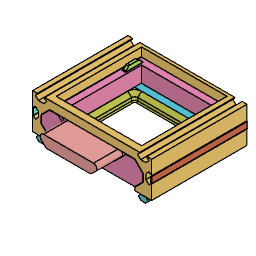
gridfinity_drawer (Autodesk Fusion 360 design; units mm, degrees)
part number: 2026-01-11-15-52-53-317
part number: 2026-01-11-15-53-28-948
part number: 2026-01-11-15-53-37-939
part number: 2026-01-11-16-03-17-954
part number: 2026-01-11-18-22-58-266
part number: 2026-01-11-18-42-20-558
part number: 2026-01-11-19-37-17-001
part number: 2026-01-13-18-50-05-171
part number: 2026-01-13-18-58-14-799
part number: 2026-01-13-19-49-23-785
part number: 2026-01-14-18-30-10-930
part number: 2026-01-14-18-30-21-173
part number: 2026-01-14-18-30-45-681
part number: 2026-01-17-12-17-04-401
part number: 2026-01-17-12-24-58-643
part number: 2026-01-17-12-34-27-194
part number: 2026-01-17-12-59-30-630
Autodesk Fusion 360 part; units mm, degrees
note: some values were not read from the file. Chosen so that the rebuilt part matches the saved one: which bodies a step acts on; that a step has no effect; a side. Set by a fixed rule: which sketch regions a step uses.
(part 1 of 2)
sketch "Schizzo1" plane through (0, 0, 0) normal (0, 0, 1) x (1, 0, 0) in component "baseplate"
  line L0 (4, 0) -> (38, 0)
  line L1 (42, 4) -> (42, 38)
  line L2 (38, 42) -> (4, 42)
  line L3 (0, 38) -> (0, 4)
  arc A0 (4, 42) -> (0, 38) centre (4, 38) ccw
  arc A1 (42, 38) -> (38, 42) centre (38, 38) ccw
  arc A2 (0, 4) -> (4, 0) centre (4, 4) ccw
  arc A3 (38, 0) -> (42, 4) centre (38, 4) ccw
  line L4 (0, 0) -> (42, 0)
  line L5 (42, 0) -> (42, 42)
  line L6 (42, 42) -> (0, 42)
  line L7 (0, 42) -> (0, 0)
  point P0 (42, 0)
  point P1 (0, 42)
  dimension "d3" = 42
  dimension "d4" = 42
  dimension "d5" = 4
  dimension "d6" = 4
  dimension "d7" = 4
  dimension "d8" = 4
  dimension "d9" = 42
  dimension "d10" = 42
  constraint horizontal L0
  constraint vertical L1
  constraint horizontal L2
  constraint vertical L3
  constraint coincident L4.start L7.end
  constraint coincident P1 L2
  constraint coincident P1 L3
  constraint tangent L2 A0
  constraint tangent L3 A0
  constraint tangent L2 A1
  constraint tangent L1 A1
  constraint coincident L4.start L3
  constraint coincident L4.start L0
  constraint tangent L3 A2
  constraint tangent L0 A2
  constraint coincident P0 L1
  constraint coincident P0 L0
  constraint tangent L1 A3
  constraint tangent L0 A3
  constraint horizontal L4
  constraint vertical L5
  constraint horizontal L6
  constraint vertical L7
  measures "d3" distance of L4.start P0
  measures "d4" distance of L4.start L6.end
  measures "d5" radius of A0
  measures "d6" radius of A1
  measures "d7" radius of A2
  measures "d8" radius of A3
  measures "d9" distance of L4.start P0
  measures "d10" distance of L4.start P1
ref_plane "Piano di lavoro1" through (21, 0, 0) normal (0, -1, 0) x (1, 0, 0) in component "baseplate"
ref_plane "Piano di lavoro2" through (21, 42, 0) normal (0, 1, 0) x (-1, 0, 0) in component "baseplate"
ref_plane "Piano di lavoro3" through (21, 21, 0) normal (0, 1, 0) x (-1, 0, 0) in component "baseplate"
sketch "Schizzo2" plane through (0, 21, 0) normal (0, 1, 0) x (1, 0, 0) in component "baseplate"
  line L0 (0, 0) -> (2.85, 0)
  line L1 (2.85, 0) -> (2.15, -0.7)
  line L2 (2.85, 0) -> (0, 0) construction
  line L3 (2.15, -0.7) -> (2.15, -2.5)
  line L4 (2.15, -2.5) -> (0, -4.65)
  line L5 (2.15, -2.5) -> (0, -2.5) construction
  line L6 (0, 0) -> (0, -4.65)
  dimension "d13" = 2.85
  dimension "d14" = 45
  dimension "d15" = 1.8
  dimension "d16" = 45
  dimension "d17" = 0.7
  dimension "d18" = 2.15
  dimension "d19" = 4.65
  constraint coincident L0.start L2.end
  constraint horizontal L0
  constraint horizontal L2
  constraint vertical L3
  constraint horizontal L5
  constraint coincident L5.end L6
  measures "d13" distance of L0.start L0.end
  measures "d14" angle of L1 L2
  measures "d15" distance of L1.end L3.end
  measures "d16" angle of L4 L5
  measures "d17" distance of L1.end L2
  measures "d18" distance of L4.end L5
  measures "d19" distance of L4.end L0.start
sweep "Sweep1" add profiles "Schizzo2" path "Schizzo1" along A2 L0 A3 L1 A1 L2 A0 L3 section 1 makes body 1 in component "baseplate"
extrude "Estrusione1" add sketch "Schizzo1" along normal blind 4.65 contours A2 L4 L7 | A3 L4 L5 | A0 L6 L7 | A1 L5 L6 bodies 1 in component "baseplate"
pattern_linear "Serie R1" [no effect] in component "baseplate"
sketch "Schizzo1 (2)" plane through (0, 0, 0) normal (0, 0, 1) x (1, 0, 0) in component "offset"
  line L0 (0, 0) -> (42, 0)
  line L1 (42, 0) -> (42, 42)
  line L2 (42, 42) -> (0, 42)
  line L3 (0, 42) -> (0, 0)
  line L4 (42.2, 46) -> (-0.2, 46)
  line L5 (42.2, 0) -> (42.2, 46)
  line L6 (-0.2, 46) -> (-0.2, 0)
  line L7 (0, 0) -> (-0.2, 0)
  line L8 (42, 0) -> (42.2, 0)
  dimension "d87" = 42
  dimension "d88" = 42
  dimension "d89" = 4
  dimension "d90" = 0.2
  dimension "d91" = 0.2
  constraint horizontal L0
  constraint vertical L1
  constraint horizontal L2
  constraint vertical L3
  constraint coincident L0.start L3.end
  constraint perpendicular L6 L7
  constraint perpendicular L5 L8
  constraint coincident L4 L6.start
  constraint coincident L4 L5.end
  constraint coincident L4.start L5
  constraint coincident L4.end L6
  measures "d87" distance of L0.start L0.end
  measures "d88" distance of L0.start L2.end
extrude "Estrusione3" add sketch "Schizzo1 (2)" along normal blind 4.65 separate body contours L1 L2 L3 L4 L5 L6 L7 L8 makes body 2 in component "offset"
sketch "Schizzo1 (3)" plane through (0, 0, 0) normal (0, 0, 1) x (1, 0, 0) in component "walls"
  line L0 (-0.2, 46) -> (42.2, 46) construction
  line L1 (42.2, 46) -> (42.2, 0) construction
  line L2 (42.2, 0) -> (-0.2, 0) construction
  line L3 (-0.2, 0) -> (-0.2, 46) construction
  line L4 (0, 46) -> (0, 0)
  line L5 (0, 46) -> (-8.8, 46)
  line L6 (-8.8, 46) -> (-8.8, 0)
  line L7 (-8.8, 0) -> (0, 0)
  line L8 (0, 0) -> (0, 46)
  line L9 (21, 46) -> (21, 0) construction
  line L10 (42, 46) -> (50.8, 46)
  line L11 (42, 0) -> (42, 46)
  line L12 (50.8, 46) -> (50.8, 0)
  line L13 (50.8, 0) -> (42, 0)
  line L14 (-8.8, 46) -> (50.8, 46)
  line L15 (50.8, 46) -> (50.8, 50)
  line L16 (50.8, 50) -> (-8.8, 50)
  line L17 (-8.8, 50) -> (-8.8, 46)
  line L18 (-0.2, 23) -> (42.2, 23) construction
  line L19 (50.8, -4) -> (-8.8, -4)
  line L20 (-8.8, -4) -> (-8.8, 0)
  line L21 (-8.8, 0) -> (50.8, 0)
  line L22 (50.8, 0) -> (50.8, -4)
  point P0 (-0.2, 46)
  point P1 (42.2, 0)
  dimension "d107" = 0.2
  dimension "d108" = 8.8
  dimension "d109" = 4
  constraint horizontal L0
  constraint vertical L1
  constraint horizontal L2
  constraint vertical L3
  constraint coincident P1 L1.end
  constraint coincident P0 L0.start
  constraint coincident L0 L4.start
  constraint perpendicular L2 L4
  constraint coincident L2 L4.end
  constraint horizontal L5
  constraint vertical L6
  constraint horizontal L7
  constraint vertical L8
  constraint midpoint L0 L9.start
  constraint midpoint L2 L9.end
  constraint symmetric L4.start L9 L10.start
  constraint symmetric L5.end L9 L10.end
  constraint symmetric L6.end L9 L12.end
  constraint symmetric L4.end L9 L11.start
  constraint horizontal L14
  constraint vertical L15
  constraint horizontal L16
  constraint vertical L17
  constraint coincident L12 L10.end
  constraint midpoint L3 L18.start
  constraint midpoint L1 L18.end
  constraint symmetric L5.end L18 L6.end
  constraint symmetric L10.end L18 L12.end
  constraint symmetric L15.end L18 L19.start
  constraint symmetric L16.end L18 L19.end
  measures "d107" distance of L3 L4
  measures "d108" distance of L4.start L5.end
  measures "d109" distance of L5.end L16.end
extrude "Estrusione1'" add sketch "Schizzo1 (3)" along normal blind 14 separate body contours L4 L5 L6 L7 L8 L14 L21 | L5 L10 L14 L15 L16 L17 | L7 L13 L19 L20 L21 L22 | L10 L11 L12 L13 L14 L21 makes body 3 in component "walls"
sketch "Schizzo2 (2)" plane through (0, -4, 0) normal (0, -1, 0) x (1, 0, 0) in component "walls"
  line L0 (-8.8, 0) -> (50.8, 0)
  line L1 (50.8, 0) -> (50.8, 14)
  line L2 (50.8, 14) -> (-8.8, 14)
  line L3 (-8.8, 14) -> (-8.8, 0)
  line L4 (21, 14) -> (21, 0) construction
  line L5 (-8.8, 7) -> (50.8, 7) construction
  line L6 (-4, 14) -> (-8.8, 9.2)
  line L7 (-4, 14) -> (-8.8, 14) construction
  line L8 (-4, 0) -> (-8.8, 4.8)
  line L9 (46, 14) -> (50.8, 9.2)
  line L10 (46, 0) -> (50.8, 4.8)
  dimension "d112" = 45
  dimension "d113" = 4.8
  constraint midpoint L2 L4.start
  constraint midpoint L0 L4.end
  constraint midpoint L3 L5.start
  constraint midpoint L1 L5.end
  constraint horizontal L7
  constraint coincident L2 L6.start
  constraint coincident L3 L6.end
  constraint coincident L3 L2.end
  constraint symmetric L5 L6.start L8.start
  constraint symmetric L5 L6.end L8.end
  constraint symmetric L4 L6.start L9.start
  constraint symmetric L4 L6.end L9.end
  constraint symmetric L4 L8.start L10.start
  constraint symmetric L4 L8.end L10.end
  measures "d112" angle of L6 L7
  measures "d113" distance of L3 L6.start
extrude "Estrusione2" cut sketch "Schizzo2 (2)" against normal up to surface (54 mm away) contours L0 L3 L8 | L0 L1 L10 | L2 L3 L6 | L1 L2 L9 bodies 3 in component "walls"
ref_plane "Piano di lavoro1" through (21, 23, 4.65) normal (0, 0, 1) x (1, 0, 0) in component "dividers"
sketch "Schizzo1 (4)" plane through (0, 0, 4.65) normal (0, 0, 1) x (1, 0, 0) in component "dividers"
  line L0 (42.2, 46) -> (-0.2, 46) construction
  line L1 (-1.8, 46) -> (0, 46)
  line L2 (0, 46) -> (0, 0)
  line L3 (0, 0) -> (-1.8, 0)
  line L4 (-1.8, 0) -> (-1.8, 46)
  line L5 (21, 46) -> (21, 34) construction
  line L6 (42, 46) -> (42, 0)
  line L7 (43.8, 46) -> (42, 46)
  line L8 (43.8, 0) -> (43.8, 46)
  line L9 (42, 0) -> (43.8, 0)
  line L10 (-1.8, 43.8) -> (43.8, 43.8)
  line L11 (43.8, 43.8) -> (43.8, 42)
  line L12 (43.8, 42) -> (-1.8, 42)
  line L13 (-1.8, 42) -> (-1.8, 43.8)
  point P0 (0, 42)
  dimension "d126" = 1.8
  dimension "d127" = 1.8
  constraint horizontal L1
  constraint vertical L2
  constraint horizontal L3
  constraint vertical L4
  constraint coincident L0 L1.end
  constraint coincident P0 L2
  constraint coincident L2.end L3.start
  constraint midpoint L0 L5.start
  constraint perpendicular L0 L5
  constraint symmetric L1.start L5 L7.start
  constraint symmetric L1.end L5 L6.start
  constraint symmetric L2.end L5 L6.end
  constraint symmetric L3.end L5 L8.start
  constraint horizontal L10
  constraint vertical L11
  constraint horizontal L12
  constraint vertical L13
  constraint coincident L4 L12.end
  constraint coincident P0 L12
  constraint coincident L8 L11.end
  measures "d126" distance of L1.start L1.end
  measures "d127" distance of L10.end L11.end
extrude "Estrusione2'" add sketch "Schizzo1 (4)" along normal blind 9.35 separate body contours L1 L2 L4 L10 | L2 L4 L10 L12 L13 | L2 L3 L4 L12 | L6 L8 L10 L11 L12 | L6 L7 L8 L10 | L6 L8 L9 L12 makes body 4 at (0, 30.6667, 7.7667) makes body 5 at (43.8, 30.6667, 10.8833) in component "dividers"
extrude "Estrusione3'" add sketch "Schizzo1 (4)" along normal blind 9.35 separate body contours L2 L6 L10 L12 makes body 6 in component "dividers"
extrude "Estrusione4" cut 1 faces at (0, 43.2, 7.7667) along direction (1, 0, 0) blind 1 on bodies 6 bodies 6 in component "dividers"
extrude "Estrusione5" cut 1 faces at (42, 43.2, 10.8833) along direction (-1, 0, 0) blind 1 on bodies 6 bodies 6 in component "dividers"
extrude "Estrusione6" add 1 faces at (1, 43.2, 7.7667) along direction (-1, 0, 0) up to surface (1 mm away) on bodies 6 bodies 6 in component "dividers"
extrude "Estrusione7" add 1 faces at (41, 43.2, 10.8833) along direction (1, 0, 0) up to surface (1 mm away) on bodies 6 bodies 6 in component "dividers"
ref_plane "Piano di lavoro1" through (21, -2, 7) normal (0, -1, 0) x (1, 0, 0) in component " handle recess"
sketch "Schizzo1 (5)" plane through (0, -2, 0) normal (0, -1, 0) x (-1, 0, 0) in component " handle recess"
  line L0 (4, -14) -> (-46, -14) construction
  line L1 (-46, -14) -> (-46, 0) construction
  line L2 (-46, 0) -> (4, 0) construction
  line L3 (4, 0) -> (4, -14) construction
  line L4 (-21, -14) -> (-21, 0) construction
  line L5 (-1, -14) -> (-7.75, -7.25)
  line L6 (-1, -14) -> (-9.2299, -14) construction
  line L7 (-41, -14) -> (-34.25, -7.25)
  line L8 (-7.75, -7.25) -> (-34.25, -7.25)
  line L9 (-41, -14) -> (-1, -14)
  line L10 (-21, -14) -> (-21, -24) construction
  line L11 (-21, -24) -> (-16, -24) construction
  line L12 (-1, -14) -> (9, -24)
  line L13 (-1, -14) -> (5.2856, -14) construction
  line L14 (-41, -14) -> (-51, -24)
  line L15 (-41, -14) -> (-49.4329, -14) construction
  point P0 (4, -14)
  point P1 (-46, 0)
  dimension "d142" = 45
  dimension "d143" = 20
  dimension "d144" = 6.75
  dimension "d145" = 10
  dimension "d146" = 5
  dimension "d147" = 45
  dimension "d148" = 45
  constraint horizontal L0
  constraint vertical L1
  constraint horizontal L2
  constraint vertical L3
  constraint coincident P1 L1.end
  constraint coincident P0 L0.start
  constraint midpoint L0 L4.start
  constraint midpoint L2 L4.end
  constraint horizontal L6
  constraint coincident L0 L5.start
  constraint symmetric L4 L5.start L7.start
  constraint symmetric L4 L5.end L7.end
  constraint perpendicular L0 L10
  constraint perpendicular L10 L11
  constraint horizontal L13
  constraint coincident L11 L12.end
  constraint horizontal L15
  constraint coincident L11 L14.end
  measures "d142" angle of L5 L6
  measures "d143" distance of L4.start L5.start
  measures "d144" distance of L5.end L6
  measures "d145" distance of L4.start L10.end
  measures "d146" distance of L10.end L11.end
  measures "d147" angle of L12 L13
  measures "d148" angle of L14 L15
ref_plane "Piano di lavoro2" through (-9, -2, 24) normal (-0.707107, 0, 0.707107) x (0, -1, 0) in component " handle recess"
sketch "Schizzo2 (3)" plane through (-9, -2, 24) normal (-0.707107, 0, 0.707107) x (0, -1, 0) in component " handle recess"
  line L0 (0.9, -2.4) -> (-0.9, -2.4)
  line L1 (-0.9, -2.4) -> (-0.9, 2.4)
  line L2 (-0.9, 2.4) -> (0.9, 2.4)
  line L3 (0.9, 2.4) -> (0.9, -2.4)
  line L4 (0.9, -2.4) -> (-0.9, 2.4) construction
  line L5 (-0.9, -2.4) -> (0.9, 2.4) construction
  dimension "d150" = 1.8
  dimension "d151" = 4.8
  constraint horizontal L0
  constraint perpendicular L0 L1
  constraint parallel L0 L2
  constraint parallel L1 L3
  constraint coincident L4 origin
  constraint coincident L5 origin
  measures "d150" distance of L1.end L2.end
  measures "d151" distance of L0.start L2.end
extrude "Estrusione3''" cut sketch "Schizzo1 (5)" along normal mid plane 4 bodies 3 in component "walls"
sweep "Sweep1'" cut profiles "Schizzo2 (3)" path "Schizzo1 (5)" along L14 L7 L8 L5 L12 section 1 bodies 3 in component "walls"
ref_plane "Piano di lavoro1" through (21, 23, 14) normal (0, 0, 1) x (1, 0, 0) in component "walls"
sketch "Schizzo3" plane through (0, 0, 14) normal (0, 0, 1) x (1, 0, 0) in component "walls"
  line L0 (-4, 50) -> (46, 50) construction
  line L1 (46, 50) -> (46, -4) construction
  line L2 (46, -4) -> (-4, -4) construction
  line L3 (-4, -4) -> (-4, 50) construction
  line L4 (21, 50) -> (21, -4) construction
  line L5 (-3, 48) -> (-1, 48)
  line L6 (-1, 48) -> (-1, 37.6)
  line L7 (-1, 37.6) -> (-3, 37.6)
  line L8 (-3, 37.6) -> (-3, 48)
  line L9 (43, 48) -> (43, 37.6)
  line L10 (45, 48) -> (43, 48)
  line L11 (45, 37.6) -> (45, 48)
  line L12 (43, 37.6) -> (45, 37.6)
  point P0 (-4, 50)
  point P1 (46, -4)
  dimension "d161" = 2
  dimension "d162" = 2
  dimension "d163" = 1
  dimension "d164" = 10.4
  constraint horizontal L0
  constraint vertical L1
  constraint horizontal L2
  constraint vertical L3
  constraint coincident P1 L1.end
  constraint coincident P0 L0.start
  constraint midpoint L0 L4.start
  constraint midpoint L2 L4.end
  constraint horizontal L5
  constraint vertical L6
  constraint horizontal L7
  constraint vertical L8
  constraint symmetric L4 L5.start L10.start
  constraint symmetric L4 L5.end L9.start
  constraint symmetric L4 L6.end L9.end
  constraint symmetric L4 L7.end L11.start
  measures "d161" distance of L0 L5
  measures "d162" distance of L5.start L5.end
  measures "d163" distance of L3 L8
  measures "d164" distance of L5.start L7.end
extrude "Estrusione4'" cut sketch "Schizzo3" against normal blind 10.4 bodies 3 in component "walls"
ref_plane "Piano di lavoro1" through (21, -1.1, 14) normal (0, -1, 0) x (-0.707107, 0, -0.707107) in component "handle"
sketch "Schizzo1 (6)" plane through (0, -1.1, 0) normal (0, -1, 0) x (-1, 0, 0) in component "handle"
  line L0 (2.3941, -14) -> (-6.7559, -4.85)
  line L1 (-6.7559, -4.85) -> (-35.2441, -4.85)
  line L2 (-35.2441, -4.85) -> (-44.3941, -14)
  line L3 (-44.3941, -14) -> (2.3941, -14)
  point P0 (2.3941, -14)
  point P1 (-6.7559, -4.85)
  point P2 (-35.2441, -4.85)
  point P3 (-44.3941, -14)
  constraint coincident P0 L0.start
  constraint coincident P1 L0.end
  constraint coincident P2 L1.end
  constraint coincident P3 L2.end
extrude "Estrusione1''" add sketch "Schizzo1 (6)" along normal blind 1.8 separate body makes body 7 in component "handle"
extrude "Estrusione6'" cut 1 faces at (13.202, -2.3, 14) along direction (0, 0, -1) blind 0.2 on bodies 7 bodies 7 in component "handle"
fillet "Raccordo2" radius 0.8 4 edges at (-2.1941, -2, 13.8) (6.7559, -2, 4.85) (35.2441, -2, 4.85) (44.1941, -2, 13.8) on bodies 7 in component "handle"
sketch "Schizzo3 (2)" plane through (0, -2.9, 0) normal (0, -1, 0) x (1, 0, 0) in component "handle"
  line L0 (-0.8284, 12.4343) -> (6.5216, 5.0843)
  line L1 (7.0873, 4.85) -> (34.9127, 4.85)
  line L2 (35.4784, 5.0843) -> (42.8284, 12.4343)
  line L3 (1, 14) -> (7.75, 7.25)
  line L4 (7.75, 7.25) -> (34.25, 7.25)
  line L5 (34.25, 7.25) -> (41, 14)
  line L6 (41, 14) -> (1, 14)
  line L7 (1.4828, 13.8) -> (7.8328, 7.45)
  line L8 (7.8328, 7.45) -> (34.1672, 7.45)
  line L9 (34.1672, 7.45) -> (40.5172, 13.8)
  line L10 (40.5172, 13.8) -> (1.4828, 13.8)
  arc A0 (42.8284, 12.4343) -> (42.2627, 13.8) centre (42.2627, 13) ccw
  line L11 (42.2627, 13.8) -> (-0.2627, 13.8)
  arc A1 (-0.2627, 13.8) -> (-0.8284, 12.4343) centre (-0.2627, 13) ccw
  arc A2 (6.5216, 5.0843) -> (7.0873, 4.85) centre (7.0873, 5.65) ccw
  arc A3 (34.9127, 4.85) -> (35.4784, 5.0843) centre (34.9127, 5.65) ccw
  point P0 (1, 14)
  point P1 (7.75, 7.25)
  point P2 (34.25, 7.25)
  point P3 (41, 14)
  dimension "d173" = -0.2
  constraint coincident P0 L3.start
  constraint coincident P1 L3.end
  constraint coincident P2 L4.end
  constraint coincident P3 L5.end
extrude "Estrusione4''" add sketch "Schizzo3 (2)" along normal blind 15 separate body contours L7 L8 L9 L10 L11 makes body 8 in component "handle"
fillet "Raccordo1" radius 2 4 edges at (1.4828, -10.4, 13.8) (7.8328, -10.4, 7.45) (34.1672, -10.4, 7.45) (40.5172, -10.4, 13.8) on bodies 8 in component "handle"
ref_plane "Piano di lavoro1" through (21, -4, 7) normal (0, -1, 0) x (1, 0, 0) in component "drawer_mount"
sketch "Schizzo1 (7)" plane through (0, -4, 0) normal (0, -1, 0) x (-1, 0, 0) in component "drawer_mount"
  line L0 (4, -14) -> (-46, -14) construction
  line L1 (-46, -14) -> (-46, 0) construction
  line L2 (-46, 0) -> (4, 0) construction
  line L3 (4, 0) -> (4, -14) construction
  line L4 (4, 0) -> (4, 2) construction
  line L5 (4, 2) -> (14, 2) construction
  line L6 (14, 2) -> (-56, 2)
  line L7 (-56, 2) -> (-56, -19)
  line L8 (-56, -19) -> (14, -19)
  line L9 (14, -19) -> (14, 2)
  point P0 (4, -14)
  point P1 (-46, 0)
  dimension "d187" = 2
  dimension "d189" = 10
  dimension "d190" = 70
  dimension "d191" = 21
  constraint horizontal L0
  constraint vertical L1
  constraint horizontal L2
  constraint vertical L3
  constraint coincident P1 L1.end
  constraint coincident P0 L0.start
  constraint perpendicular L2 L4
  constraint perpendicular L4 L5
  constraint horizontal L6
  constraint vertical L7
  constraint horizontal L8
  constraint vertical L9
  measures "d187" distance of L2.end L4.end
  measures "d189" distance of L4.end L5.end
  measures "d190" distance of L5.end L6.end
  measures "d191" distance of L5.end L8.end
extrude "Estrusione1'''" add sketch "Schizzo1 (7)" against normal blind 56 separate body makes body 9 in component "drawer_mount"
sketch "Schizzo2 (4)" plane through (0, -4, 0) normal (0, -1, 0) x (1, 0, 0) in component "drawer_mount"
  line L0 (-14, 19) -> (-14, -2)
  line L1 (-14, -2) -> (56, -2)
  line L2 (56, -2) -> (56, 19)
  line L3 (56, 19) -> (-14, 19)
  line L4 (-4, 14) -> (46, 14) construction
  line L5 (46, 14) -> (46, 0) construction
  line L6 (46, 0) -> (-4, 0) construction
  line L7 (-4, 0) -> (-4, 14) construction
  line L8 (-4, 14) -> (-8.8, 9.2) construction
  line L9 (-8.8, 4.8) -> (-8.8, 9.2) construction
  line L10 (-8.8, 4.8) -> (-4, 0) construction
  line L11 (46, 0) -> (50.8, 4.8) construction
  line L12 (50.8, 4.8) -> (50.8, 9.2) construction
  line L13 (50.8, 9.2) -> (46, 14) construction
  line L14 (-4.0828, 14.2) -> (-9, 9.2828)
  line L15 (-9, 4.7172) -> (-9, 9.2828)
  line L16 (-9, 4.7172) -> (-4.0828, -0.2)
  line L17 (46.0828, -0.2) -> (-4.0828, -0.2)
  line L18 (46.0828, -0.2) -> (51, 4.7172)
  line L19 (51, 4.7172) -> (51, 9.2828)
  line L20 (51, 9.2828) -> (46.0828, 14.2)
  line L21 (-4.0828, 14.2) -> (46.0828, 14.2)
  line L22 (-4.0828, -0.2) -> (-4.0828, -2)
  line L23 (46.0828, -0.2) -> (46.0828, -2)
  point P0 (-4, 14)
  point P1 (46, 0)
  dimension "d194" = -0.2
  constraint horizontal L4
  constraint vertical L5
  constraint horizontal L6
  constraint vertical L7
  constraint coincident P1 L5.end
  constraint coincident P0 L4.start
  constraint coincident L1 L22.end
  constraint perpendicular L1 L22
  constraint perpendicular L1 L23
  constraint coincident L1 L23.end
extrude "Estrusione2''" cut sketch "Schizzo2 (4)" against normal up to surface (54.2 mm away) contours L1 L17 L22 L23 | L14 L15 L16 L17 L18 L19 L20 L21 bodies 9 in component "drawer_mount"
sketch "Schizzo3 (3)" plane through (0, 0, 19) normal (0, 0, 1) x (-1, 0, 0) in component "drawer_mount"
  line L0 (14, 4) -> (-56, 4)
  line L1 (-56, 4) -> (-56, -52)
  line L2 (-56, -52) -> (14, -52)
  line L3 (14, -52) -> (14, 4)
  line L4 (4.0828, 4) -> (4.0828, -50.2) construction
  line L5 (-46.0828, 4) -> (-46.0828, -50.2) construction
  line L6 (4.0828, -50.2) -> (-46.0828, -50.2)
  line L7 (-46.0828, -50.2) -> (-46.0828, 0)
  line L8 (-46.0828, 0) -> (4.0828, 0)
  line L9 (4.0828, 0) -> (4.0828, -50.2)
  dimension "d197" = 4
  constraint horizontal L6
  constraint vertical L7
  constraint horizontal L8
  constraint vertical L9
  constraint coincident L4 L8.end
  constraint coincident L5 L7.end
  constraint coincident L4.end L6.start
  measures "d197" distance of L0 L8
extrude "Estrusione3'''" cut sketch "Schizzo3 (3)" against normal up to surface (4.8 mm away) contours L6 L7 L8 L9 bodies 9 in component "drawer_mount"
ref_plane "Piano di lavoro2" through (21, -4, 8.5) normal (0, -1, 0) x (-1, 0, 0) in component "drawer_mount"
sketch "Schizzo5" plane through (0, -4, 0) normal (0, -1, 0) x (-1, 0, 0) in component "drawer_mount"
  line L0 (14, -19) -> (-56, -19) construction
  line L1 (-56, -19) -> (-56, 2) construction
  line L2 (-56, 2) -> (14, 2) construction
  line L3 (14, 2) -> (14, -19) construction
  line L4 (-21, 2) -> (-21, -2) construction
  line L5 (14, -6.4) -> (13.6, -6.4)
  line L6 (13.6, -6.4) -> (12.4, -5.2)
  line L7 (13.6, -6.4) -> (14, -6.4) construction
  line L8 (12.4, -5.2) -> (10.6, -7)
  line L9 (12.4, -5.2) -> (14, -5.2) construction
  line L10 (10.6, -7) -> (10.6, -8.5)
  line L11 (10.6, -8.5) -> (14, -8.5) construction
  line L12 (14, -10.6) -> (13.6, -10.6)
  line L13 (13.6, -10.6) -> (12.4, -11.8)
  line L14 (12.4, -11.8) -> (10.6, -10)
  line L15 (10.6, -10) -> (10.6, -8.5)
  line L16 (14, -10.6) -> (14, -6.4)
  line L17 (-56, -10.6) -> (-56, -6.4)
  line L18 (-56, -10.6) -> (-55.6, -10.6)
  line L19 (-55.6, -10.6) -> (-54.4, -11.8)
  line L20 (-54.4, -11.8) -> (-52.6, -10)
  line L21 (-52.6, -10) -> (-52.6, -8.5)
  line L22 (-52.6, -7) -> (-52.6, -8.5)
  line L23 (-54.4, -5.2) -> (-52.6, -7)
  line L24 (-55.6, -6.4) -> (-54.4, -5.2)
  line L25 (-56, -6.4) -> (-55.6, -6.4)
  line L26 (-21, -19) -> (-21, -16) construction
  line L27 (11.141, -19) -> (11.141, -18.6)
  line L28 (11.141, -18.6) -> (12.341, -17.4)
  line L29 (11.141, -18.6) -> (9.041, -18.6) construction
  line L30 (12.341, -17.4) -> (10.541, -15.6)
  line L31 (12.341, -17.4) -> (9.041, -17.4) construction
  line L32 (10.541, -15.6) -> (9.041, -15.6)
  line L33 (9.041, -15.6) -> (9.041, -19) construction
  line L34 (6.941, -19) -> (6.941, -18.6)
  line L35 (6.941, -18.6) -> (5.741, -17.4)
  line L36 (5.741, -17.4) -> (7.541, -15.6)
  line L37 (7.541, -15.6) -> (9.041, -15.6)
  line L38 (6.941, -19) -> (11.141, -19)
  line L39 (9.041, -15.6) -> (9.041, 2) construction
  line L40 (11.141, 2) -> (11.141, 2.4) construction
  line L41 (11.141, 2.4) -> (12.341, 3.6) construction
  line L42 (11.141, 2.4) -> (9.041, 2.4) construction
  line L43 (12.341, 3.6) -> (10.541, 5.4) construction
  line L44 (12.341, 3.6) -> (9.041, 3.6) construction
  line L45 (10.541, 5.4) -> (9.041, 5.4) construction
  line L46 (6.941, 2) -> (6.941, 2.4) construction
  line L47 (6.941, 2.4) -> (5.741, 3.6) construction
  line L48 (5.741, 3.6) -> (7.541, 5.4) construction
  line L49 (7.541, 5.4) -> (9.041, 5.4) construction
  line L50 (10.941, 2) -> (10.941, 2.4828)
  line L51 (10.941, 2.4828) -> (12.0582, 3.6)
  line L52 (12.0582, 3.6) -> (10.4582, 5.2)
  line L53 (10.4582, 5.2) -> (44.041, 5.2)
  line L54 (7.6238, 5.2) -> (44.041, 5.2)
  line L55 (6.0238, 3.6) -> (7.6238, 5.2)
  line L56 (7.141, 2.4828) -> (6.0238, 3.6)
  line L57 (7.141, 2) -> (7.141, 2.4828)
  line L58 (10.941, 2) -> (7.141, 2)
  line L59 (-52.941, 2) -> (-49.141, 2)
  line L60 (-52.941, 2) -> (-52.941, 2.4828)
  line L61 (-52.941, 2.4828) -> (-54.0582, 3.6)
  line L62 (-54.0582, 3.6) -> (-52.4582, 5.2)
  line L63 (-52.4582, 5.2) -> (-86.041, 5.2)
  line L64 (-49.6238, 5.2) -> (-86.041, 5.2)
  line L65 (-48.0238, 3.6) -> (-49.6238, 5.2)
  line L66 (-49.141, 2.4828) -> (-48.0238, 3.6)
  line L67 (-49.141, 2) -> (-49.141, 2.4828)
  line L68 (-48.941, -19) -> (-53.141, -19)
  line L69 (-53.141, -19) -> (-53.141, -18.6)
  line L70 (-53.141, -18.6) -> (-54.341, -17.4)
  line L71 (-54.341, -17.4) -> (-52.541, -15.6)
  line L72 (-52.541, -15.6) -> (-51.041, -15.6)
  line L73 (-49.541, -15.6) -> (-51.041, -15.6)
  line L74 (-47.741, -17.4) -> (-49.541, -15.6)
  line L75 (-48.941, -18.6) -> (-47.741, -17.4)
  line L76 (-48.941, -19) -> (-48.941, -18.6)
  point P0 (14, -19)
  point P1 (-56, 2)
  dimension "d201" = 0.4
  dimension "d202" = 45
  dimension "d203" = 45
  dimension "d204" = 1.5
  dimension "d205" = 10.5
  dimension "d206" = 1.2
  dimension "d207" = 1.8
  dimension "d208" = 35
  dimension "d209" = 0.4
  dimension "d210" = 45
  dimension "d211" = 45
  dimension "d212" = 1.5
  dimension "d213" = 4.959
  dimension "d214" = 1.2
  dimension "d215" = 1.8
  dimension "d216" = 0.4
  dimension "d217" = 45
  dimension "d218" = 45
  dimension "d219" = 1.5
  dimension "d220" = 1.2
  dimension "d221" = 1.8
  dimension "d222" = 0.2
  constraint horizontal L0
  constraint vertical L1
  constraint horizontal L2
  constraint vertical L3
  constraint coincident P1 L1.end
  constraint coincident P0 L0.start
  constraint midpoint L2 L4.start
  constraint perpendicular L2 L4
  constraint coincident L3 L5.start
  constraint perpendicular L3 L5
  constraint horizontal L7
  constraint horizontal L9
  constraint vertical L10
  constraint coincident L3 L11.end
  constraint perpendicular L3 L11
  constraint symmetric L5.start L11 L12.start
  constraint symmetric L5.end L11 L12.end
  constraint symmetric L6.end L11 L13.end
  constraint symmetric L8.end L11 L14.end
  constraint symmetric L10.end L11 L15.end
  constraint symmetric L4 L5.start L17.end
  constraint symmetric L4 L5.end L24.start
  constraint symmetric L4 L6.end L23.start
  constraint symmetric L4 L8.end L22.start
  constraint symmetric L4 L10.end L21.end
  constraint symmetric L4 L12.start L17.start
  constraint symmetric L4 L12.end L18.end
  constraint symmetric L4 L13.end L19.end
  constraint symmetric L4 L14.end L20.end
  constraint coincident L3 L9.end
  constraint coincident L0 L26.start
  constraint perpendicular L0 L26
  constraint coincident L0 L27.start
  constraint perpendicular L0 L27
  constraint horizontal L29
  constraint horizontal L31
  constraint horizontal L32
  constraint coincident L0 L33.end
  constraint perpendicular L32 L33
  constraint coincident L31.end L33
  constraint coincident L29.end L33
  constraint symmetric L27.start L33 L34.start
  constraint symmetric L27.end L33 L34.end
  constraint symmetric L28.end L33 L35.end
  constraint symmetric L30.end L33 L36.end
  constraint symmetric L32.end L33 L37.end
  constraint perpendicular L2 L39
  constraint coincident L2 L39.end
  constraint coincident L2 L40.start
  constraint perpendicular L2 L40
  constraint horizontal L42
  constraint horizontal L44
  constraint horizontal L45
  constraint coincident L39 L45.end
  constraint symmetric L39 L40.start L46.start
  constraint symmetric L39 L40.end L46.end
  constraint symmetric L39 L41.end L47.end
  constraint symmetric L39 L43.end L48.end
  constraint symmetric L39 L45.end L49.end
  constraint coincident L39 L44.end
  constraint coincident L39 L42.end
  constraint coincident L2 L50.start
  constraint coincident L2 L57.start
  constraint symmetric L4 L50.start L59.start
  constraint symmetric L4 L50.end L60.end
  constraint symmetric L4 L51.end L61.end
  constraint symmetric L4 L52.end L62.end
  constraint symmetric L4 L53.end L63.end
  constraint symmetric L4 L54.start L64.start
  constraint symmetric L4 L55.start L65.start
  constraint symmetric L4 L56.start L66.start
  constraint symmetric L4 L57.start L59.end
  constraint symmetric L26 L27.start L68.end
  constraint symmetric L26 L27.end L69.end
  constraint symmetric L26 L28.end L70.end
  constraint symmetric L26 L30.end L71.end
  constraint symmetric L26 L32.end L72.end
  constraint symmetric L26 L34.start L68.start
  constraint symmetric L26 L34.end L75.start
  constraint symmetric L26 L35.end L74.start
  constraint symmetric L26 L36.end L73.start
  measures "d201" distance of L5.start L5.end
  measures "d202" angle of L6 L7
  measures "d203" angle of L8 L9
  measures "d204" distance of L8.end L10.end
  measures "d205" distance of L2.end L11.end
  measures "d206" horizontal distance of L5.end L6.end
  measures "d207" horizontal distance of L6.end L8.end
  measures "d208" distance of P0 L26.start
  measures "d209" distance of L27.start L27.end
  measures "d210" angle of L28 L29
  measures "d211" angle of L30 L31
  measures "d212" distance of L30.end L32.end
  measures "d213" distance of P0 L33.end
  measures "d214" vertical distance of L27.end L28.end
  measures "d215" vertical distance of L28.end L30.end
  measures "d216" distance of L40.start L40.end
  measures "d217" angle of L41 L42
  measures "d218" angle of L43 L44
  measures "d219" distance of L43.end L45.end
  measures "d220" vertical distance of L40.end L41.end
  measures "d221" vertical distance of L41.end L43.end
extrude "Estrusione1''''" add sketch "Schizzo5" against normal up to surface (56 mm away) separate body contours L50 L51 L52 L54 L55 L56 L57 L58 | L59 L60 L61 L62 L64 L65 L66 L67 makes body 10 at (-8.4077, 33.3333, -2) makes body 11 at (51.6743, 14.6667, -2) in component "foots"
extrude "Estrusione4'''" cut sketch "Schizzo5" against normal up to surface (56 mm away) contours L5 L6 L8 L10 L12 L13 L14 L15 L16 | L17 L18 L19 L20 L21 L22 L23 L24 L25 bodies 9 in component "drawer_mount"
pattern_linear "Serie R1'" [no effect] in component "drawer_mount"
extrude "Estrusione6''" cut sketch "Schizzo5" against normal up to surface (56 mm away) contours L27 L28 L30 L32 L34 L35 L36 L37 L38 | L68 L69 L70 L71 L72 L73 L74 L75 L76 bodies 9 in component "drawer_mount"
pattern_linear "Serie R2" [no effect] in component "drawer_mount"
ref_plane "Piano di lavoro1" through (-13.8, 24, 6.4) normal (0, 0, 1) x (1, 0, 0) in component "spots"
sketch "Schizzo1 (8)" plane through (0, 0, 6.4) normal (0, 0, 1) x (1, 0, 0) in component "spots"
  line L0 (-14, -3.6) -> (-13.6, -3.6)
  line L1 (-13.6, -3.6) -> (-13.6, -4)
  line L2 (-13.6, -4) -> (-14, -4)
  line L3 (-14, -4) -> (-14, -3.6)
  point P0 (-14, -4)
  point P1 (-13.6, -4)
  dimension "d263" = 0.4
  constraint horizontal L0
  constraint vertical L1
  constraint horizontal L2
  constraint vertical L3
  constraint coincident P0 L2.end
  constraint coincident P1 L1.end
  measures "d263" distance of L0.start P0
extrude "Estrusione1'''''" add sketch "Schizzo1 (8)" along normal blind 0.2 separate body makes body 12 in component "spots"
ref_plane "Piano di lavoro2" through (-13.8, 24, 8.5) normal (0, 0, 1) x (1, 0, 0) in component "spots"
mirror "Specchio1" about plane through (-13.8, 24, 8.5) normal (0, 0, 1) of bodies 12 makes body 13 in component "spots"
pattern_linear "Serie R1''" count 18 spacing 3.2706 along (0, 1, 0) of bodies 12 13 makes body 14 at (-13.8667, -0.5961, 6.4) makes body 15 at (-13.8667, 2.6745, 6.4) makes body 16 at (-13.8667, 5.9451, 6.4) makes body 17 at (-13.8667, 9.2157, 6.4) makes body 18 at (-13.8667, 12.4863, 6.4) makes body 19 at (-13.8667, 15.7569, 6.4) makes body 20 at (-13.8667, 19.0275, 6.4) makes body 21 at (-13.8667, 22.298, 6.4) makes body 22 at (-13.8667, 25.5686, 6.4) makes body 23 at (-13.8667, 28.8392, 6.4) makes body 24 at (-13.8667, 32.2431, 6.4) makes body 25 at (-13.8667, 35.5137, 6.4) makes body 26 at (-13.8667, 38.7843, 6.4) makes body 27 at (-13.8667, 42.0549, 6.4) makes body 28 at (-13.8667, 45.3255, 6.4) makes body 29 at (-13.8667, 48.5961, 6.4) makes body 30 at (-13.8667, 51.8667, 6.4) makes body 31 at (-13.8667, -0.5961, 10.6) makes body 32 at (-13.8667, 2.6745, 10.6) makes body 33 at (-13.8667, 5.9451, 10.6) makes body 34 at (-13.8667, 9.2157, 10.6) makes body 35 at (-13.8667, 12.4863, 10.6) makes body 36 at (-13.8667, 15.7569, 10.6) makes body 37 at (-13.8667, 19.0275, 10.6) makes body 38 at (-13.8667, 22.298, 10.6) makes body 39 at (-13.8667, 25.5686, 10.6) makes body 40 at (-13.8667, 28.8392, 10.6) makes body 41 at (-13.8667, 32.2431, 10.6) makes body 42 at (-13.8667, 35.5137, 10.6) makes body 43 at (-13.8667, 38.7843, 10.6) makes body 44 at (-13.8667, 42.0549, 10.6) makes body 45 at (-13.8667, 45.3255, 10.6) makes body 46 at (-13.8667, 48.5961, 10.6) makes body 47 at (-13.8667, 51.8667, 10.6) in component "spots"
ref_plane "Piano di lavoro1" through (-13.8, 24, 6.6) normal (0, 0, 1) x (1, 0, 0) in component "left"
sketch "Schizzo1 (9)" plane through (0, 0, 6.6) normal (0, 0, 1) x (1, 0, 0) in component "left"
  line L0 (-13.6, 52) -> (-14, 52)
  line L1 (-14, 52) -> (-14, -4)
  line L2 (-14, -4) -> (-13.6, -4)
  line L3 (-13.6, -4) -> (-13.6, 52)
  point P0 (-14, -4)
  point P1 (-13.6, 52)
  constraint horizontal L0
  constraint vertical L1
  constraint horizontal L2
  constraint vertical L3
  constraint coincident P0 L1.end
  constraint coincident P1 L0.start
extrude "Estrusione1''''''" add sketch "Schizzo1 (9)" along normal up to surface (3.8 mm away) separate body makes body 48 in component "left"
extrude "Estrusione2'''" add 1 faces at (-14, 33.3333, 7.8667) along direction (-1, 0, 0) blind 0.1 on bodies 48 bodies 48 in component "left"
extrude "Estrusione3''''" add 1 faces at (-13.6, 14.6667, 7.8667) along direction (1, 0, 0) blind 0.1 on bodies 48 bodies 48 in component "left"
chamfer "Smusso1" distance 0.1 angle 45 2 edges at (-14.1, 24, 6.6) (-13.5, 24, 6.6) on bodies 48 in component "left"
chamfer "Smusso2" distance 0.1 angle 45 2 edges at (-14.1, 24, 10.4) (-13.5, 24, 10.4) on bodies 48 in component "left"
ref_plane "Piano di lavoro1" through (21, 24, 8.5) normal (-1, 0, 0) x (0, 0, 1) in component "supports"
mirror "SpecchiaComponente1" about plane through (0, 0, 0) normal (0, 0, 1) of bodies 48 makes body 49 in component "right"
mirror "SpecchiaComponente1'" about plane through (0, 0, 0) normal (0, 0, 1) of bodies 12 13 14 15 16 17 18 19 20 21 22 23 24 25 26 27 28 29 30 31 32 33 34 35 36 37 38 39 40 41 42 43 44 45 46 47 makes body 50 at (-13.8667, -3.8667, -6.4) makes body 51 at (-13.8667, -3.8667, -10.6) makes body 52 at (-13.8667, -0.5961, -6.4) makes body 53 at (-13.8667, 2.6745, -6.4) makes body 54 at (-13.8667, 5.9451, -6.4) makes body 55 at (-13.8667, 9.2157, -6.4) makes body 56 at (-13.8667, 12.4863, -6.4) makes body 57 at (-13.8667, 15.7569, -6.4) makes body 58 at (-13.8667, 19.0275, -6.4) makes body 59 at (-13.8667, 22.298, -6.4) makes body 60 at (-13.8667, 25.5686, -6.4) makes body 61 at (-13.8667, 28.8392, -6.4) makes body 62 at (-13.8667, 32.2431, -6.4) makes body 63 at (-13.8667, 35.5137, -6.4) makes body 64 at (-13.8667, 38.7843, -6.4) makes body 65 at (-13.8667, 42.0549, -6.4) makes body 66 at (-13.8667, 45.3255, -6.4) makes body 67 at (-13.8667, 48.5961, -6.4) makes body 68 at (-13.8667, 51.8667, -6.4) makes body 69 at (-13.8667, -0.5961, -10.6) makes body 70 at (-13.8667, 2.6745, -10.6) makes body 71 at (-13.8667, 5.9451, -10.6) makes body 72 at (-13.8667, 9.2157, -10.6) makes body 73 at (-13.8667, 12.4863, -10.6) makes body 74 at (-13.8667, 15.7569, -10.6) makes body 75 at (-13.8667, 19.0275, -10.6) makes body 76 at (-13.8667, 22.298, -10.6) makes body 77 at (-13.8667, 25.5686, -10.6) makes body 78 at (-13.8667, 28.8392, -10.6) makes body 79 at (-13.8667, 32.2431, -10.6) makes body 80 at (-13.8667, 35.5137, -10.6) makes body 81 at (-13.8667, 38.7843, -10.6) makes body 82 at (-13.8667, 42.0549, -10.6) makes body 83 at (-13.8667, 45.3255, -10.6) makes body 84 at (-13.8667, 48.5961, -10.6) makes body 85 at (-13.8667, 51.8667, -10.6) in component "spots(Specchio)"
pattern_linear "Serie R1'''" [suppressed] in component "supports"
ref_plane "Piano di lavoro1" through (21, -4, 8.5) normal (0, -1, 0) x (-1, 0, 0) in component "top_cover"
sketch "Schizzo1 (10)" plane through (0, -4, 0) normal (0, -1, 0) x (-1, 0, 0) in component "top_cover"
  line L0 (14, -19) -> (-56, -19) construction
  line L1 (-56, -19) -> (-56, 2) construction
  line L2 (-56, 2) -> (14, 2) construction
  line L3 (14, 2) -> (14, -19) construction
  line L4 (11.141, -19) -> (11.141, -18.6)
  line L5 (11.141, -18.6) -> (12.341, -17.4)
  line L6 (11.141, -18.6) -> (10.4, -18.6) construction
  line L7 (12.341, -17.4) -> (10.541, -15.6)
  line L8 (12.341, -17.4) -> (11.1337, -17.4) construction
  line L9 (10.541, -15.6) -> (9.041, -15.6)
  line L10 (9.041, -15.6) -> (9.041, -19) construction
  line L11 (6.941, -19) -> (6.941, -18.6)
  line L12 (6.941, -18.6) -> (5.741, -17.4)
  line L13 (5.741, -17.4) -> (7.541, -15.6)
  line L14 (7.541, -15.6) -> (9.041, -15.6)
  line L15 (10.941, -19) -> (10.941, -18.5172)
  line L16 (10.941, -18.5172) -> (12.0582, -17.4)
  line L17 (12.0582, -17.4) -> (10.4582, -15.8)
  line L18 (10.4582, -15.8) -> (9.041, -15.8)
  line L19 (7.6238, -15.8) -> (9.041, -15.8)
  line L20 (6.0238, -17.4) -> (7.6238, -15.8)
  line L21 (7.141, -18.5172) -> (6.0238, -17.4)
  line L22 (7.141, -19) -> (7.141, -18.5172)
  line L23 (14, -19) -> (-56, -19)
  line L24 (-56, -19) -> (-56, -20.8)
  line L25 (-56, -20.8) -> (14, -20.8)
  line L26 (14, -20.8) -> (14, -19)
  line L27 (-21, -19) -> (-21, -15) construction
  line L28 (-52.941, -19) -> (-52.941, -18.5172)
  line L29 (-52.941, -18.5172) -> (-54.0582, -17.4)
  line L30 (-54.0582, -17.4) -> (-52.4582, -15.8)
  line L31 (-52.4582, -15.8) -> (-51.041, -15.8)
  line L32 (-49.6238, -15.8) -> (-51.041, -15.8)
  line L33 (-48.0238, -17.4) -> (-49.6238, -15.8)
  line L34 (-49.141, -18.5172) -> (-48.0238, -17.4)
  line L35 (-49.141, -19) -> (-49.141, -18.5172)
  point P0 (14, -19)
  point P1 (-56, 2)
  point P2 (11.141, -19)
  dimension "d288" = 0.4
  dimension "d289" = 45
  dimension "d290" = 45
  dimension "d291" = 1.5
  dimension "d292" = 1.2
  dimension "d293" = 1.8
  dimension "d294" = 0.2
  dimension "d295" = 1.8
  dimension "d296" = 35
  constraint horizontal L0
  constraint vertical L1
  constraint horizontal L2
  constraint vertical L3
  constraint coincident P1 L1.end
  constraint coincident P0 L0.start
  constraint coincident L0 P2
  constraint perpendicular L0 L4
  constraint horizontal L6
  constraint horizontal L8
  constraint horizontal L9
  constraint coincident P2 L4.start
  constraint coincident L0 L10.end
  constraint perpendicular L0 L10
  constraint symmetric P2 L10 L11.start
  constraint symmetric L4.end L10 L11.end
  constraint symmetric L5.end L10 L12.end
  constraint symmetric L7.end L10 L13.end
  constraint symmetric L9.end L10 L14.end
  constraint horizontal L23
  constraint vertical L24
  constraint horizontal L25
  constraint vertical L26
  constraint coincident L0.end L1.start
  constraint coincident L0 L27.start
  constraint perpendicular L0 L27
  constraint coincident L15.start L23
  constraint coincident L0 L22.start
  constraint symmetric L15.start L27 L28.start
  constraint symmetric L15.end L27 L28.end
  constraint symmetric L16.end L27 L29.end
  constraint symmetric L17.end L27 L30.end
  constraint symmetric L18.end L27 L31.end
  constraint symmetric L19.start L27 L32.start
  constraint symmetric L20.start L27 L33.start
  constraint symmetric L21.start L27 L34.start
  constraint symmetric L22.start L27 L35.start
  measures "d288" distance of P2 L4.end
  measures "d289" angle of L5 L6
  measures "d290" angle of L7 L8
  measures "d291" distance of L7.end L9.end
  measures "d292" distance of L5.end L6
  measures "d293" distance of L7.end L8
  measures "d295" distance of P0 L25.end
  measures "d296" distance of L3 L27
extrude "Estrusione1'''''''" add sketch "Schizzo1 (10)" against normal up to surface (56 mm away) separate body contours L23 L24 L25 L26 makes body 86 in component "top_cover"
extrude "Estrusione1''''''''" add sketch "Schizzo1 (10)" against normal up to surface (56 mm away) separate body contours L15 L16 L17 L18 L19 L20 L21 L22 L23 | L23 L28 L29 L30 L31 L32 L33 L34 L35 makes body 87 at (-8.4077, 33.3333, 19) makes body 88 at (50.4077, 14.6667, 19) in component "tracks"
pattern_linear "Serie R1''''" [suppressed] in component "top_cover"
ref_plane "Piano di lavoro1" through (21, 24, 19) normal (0, 0, 1) x (1, 0, 0) in component "top_mount_holes"
sketch "Schizzo1 (11)" plane through (0, 0, 19) normal (0, 0, 1) x (1, 0, 0) in component "top_mount_holes"
  line L0 (-4.0828, 50.2) -> (46.0828, 50.2) construction
  line L1 (46.0828, 50.2) -> (46.0828, 0) construction
  line L2 (46.0828, 0) -> (-4.0828, 0) construction
  line L3 (-4.0828, 0) -> (-4.0828, 50.2) construction
  line L4 (21, 50.2) -> (21, 0) construction
  line L5 (-4.0828, 25.1) -> (46.0828, 25.1) construction
  line L6 (-4.0828, 50.2) -> (9.9172, 50.2)
  line L7 (9.9172, 50.2) -> (9.9172, 36.2)
  line L8 (9.9172, 36.2) -> (-4.0828, 36.2)
  line L9 (-4.0828, 36.2) -> (-4.0828, 50.2)
  line L10 (32.0828, 36.2) -> (46.0828, 36.2)
  line L11 (32.0828, 50.2) -> (32.0828, 36.2)
  line L12 (46.0828, 50.2) -> (32.0828, 50.2)
  line L13 (46.0828, 36.2) -> (46.0828, 50.2)
  line L14 (-4.0828, 0) -> (9.9172, 0)
  line L15 (9.9172, 0) -> (9.9172, 14)
  line L16 (-4.0828, 14) -> (-4.0828, 0)
  line L17 (9.9172, 14) -> (-4.0828, 14)
  line L18 (46.0828, 14) -> (46.0828, 0)
  line L19 (46.0828, 0) -> (32.0828, 0)
  line L20 (32.0828, 0) -> (32.0828, 14)
  line L21 (32.0828, 14) -> (46.0828, 14)
  point P0 (-4.0828, 50.2)
  point P1 (46.0828, 0)
  dimension "d309" = 14
  dimension "d310" = 14
  constraint horizontal L0
  constraint vertical L1
  constraint horizontal L2
  constraint vertical L3
  constraint coincident P1 L1.end
  constraint coincident P0 L0.start
  constraint midpoint L0 L4.start
  constraint midpoint L2 L4.end
  constraint midpoint L3 L5.start
  constraint midpoint L1 L5.end
  constraint horizontal L6
  constraint vertical L7
  constraint horizontal L8
  constraint vertical L9
  constraint symmetric P0 L4 L0.end
  constraint symmetric L4 L6.end L11.start
  constraint symmetric L4 L7.end L10.start
  constraint symmetric L4 L8.end L10.end
  constraint symmetric P0 L5 L2.end
  constraint symmetric L5 L6.end L14.end
  constraint symmetric L5 L7.end L15.end
  constraint symmetric L5 L8.end L16.start
  constraint symmetric L5 L10.start L20.end
  constraint symmetric L5 L10.end L18.start
  constraint symmetric L5 L11.start L19.end
  constraint symmetric L5 L0.end P1
  measures "d309" distance of L6.end L7.end
  measures "d310" distance of L7.end L8.end
extrude "Estrusione1'''''''''" add sketch "Schizzo1 (11)" against normal blind 2.25 separate body makes body 89 at (41.4162, 40.8667, 19) makes body 90 at (41.4162, 9.3333, 19) makes body 91 at (0.5838, 40.8667, 19) makes body 92 at (0.5838, 9.3333, 19) in component "top_mount_holes"
ref_plane "Piano di lavoro2" through (2.9172, 7, 16.75) normal (0, 0, -1) x (-1, 0, 0) in component "top_mount_holes"
sketch "Schizzo2 (5)" plane through (0, 0, 16.75) normal (0, 0, -1) x (-1, 0, 0) in component "top_mount_holes"
  line L0 (4.0828, 50.2) -> (-46.0828, 50.2) construction
  line L1 (-46.0828, 50.2) -> (-46.0828, 0) construction
  line L2 (-46.0828, 0) -> (4.0828, 0) construction
  line L3 (4.0828, 0) -> (4.0828, 50.2) construction
  line L4 (-21, 50.2) -> (-21, 0) construction
  line L5 (-46.0828, 25.1) -> (4.0828, 25.1) construction
  line L6 (4.0828, 50.2) -> (-9.9172, 36.2) construction
  line L7 (4.0828, 36.2) -> (-9.9172, 50.2) construction
  point P0 (4.0828, 50.2)
  point P1 (-46.0828, 0)
  point P2 (-9.9172, 36.2)
  point P3 (-9.9172, 50.2)
  point P4 (4.0828, 36.2)
  point P5 (-2.9172, 43.2)
  point P6 (-39.0828, 43.2)
  point P7 (-2.9172, 7)
  point P8 (-39.0828, 7)
  constraint horizontal L0
  constraint vertical L1
  constraint horizontal L2
  constraint vertical L3
  constraint coincident P1 L1.end
  constraint coincident P0 L0.start
  constraint midpoint L0 L4.start
  constraint midpoint L2 L4.end
  constraint midpoint L1 L5.start
  constraint midpoint L3 L5.end
  constraint coincident P2 L6.end
  constraint coincident P4 L7.start
  constraint coincident P3 L7.end
  constraint midpoint L7 P5
  constraint symmetric L4 P5 P6
  constraint symmetric L5 P5 P7
  constraint symmetric L5 P6 P8
hole "Foratura1" at (39.0828, 43.2, 16.75) at (2.9172, 43.2, 16.75) at (39.0828, 7, 16.75) at (2.9172, 7, 16.75) direction (0, 0, 1) diameter 3.5 depth 16 tip angle 118 countersink diameter 6 countersink angle 90 bodies 89 90 91 92 in component "top_mount_holes"
fillet "Raccordo1'" radius 4 4 edges at (32.0828, 36.2, 17.875) (32.0828, 14, 17.875) (9.9172, 36.2, 17.875) (9.9172, 14, 17.875) on bodies 89 90 91 92 in component "top_mount_holes"
ref_plane "Piano di lavoro1" through (-2.8, 42.8, 8.8) normal (1, 0, 0) x (0, -1, 0) in component "spring"